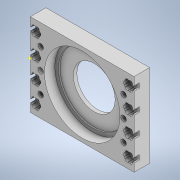
# Autodesk Inventor part: BearingBlock
Saved by Autodesk Inventor 2020 (Build 240168000, 168)
## iProperties
Created: 2020-01-26
Part Number: BearingBlock
Material: Generic
Document SubType Name: Modeling
Designer: srini
Density: 1 g/cm^3
Appearance: Default
Author: srini
Autodesk Inventor part; units mm, degrees
ref_plane "YZ Plane" through (0, 0, 0) normal (1, 0, 0) x (0, 1, 0)
ref_plane "XZ Plane" through (0, 0, 0) normal (0, 1, 0) x (-1, 0, 0)
ref_plane "XY Plane" through (0, 0, 0) normal (0, 0, 1) x (1, 0, 0)
sketch "Sketch1" plane through (0, 0, 0) normal (1, 0, 0) x (0, 1, 0)
  line L0 (43.9796, 9.0546) -> (-57.6204, 9.0546)
  line L1 (-57.6204, 9.0546) -> (-57.6204, -9.9954)
  line L2 (-57.6204, -9.9954) -> (43.9796, -9.9954)
  line L3 (43.9796, -9.9954) -> (43.9796, 9.0546)
  point P0 (0, 0)
  dimension "d0" = 19.05
  dimension "d1" = 101.6
  constraints: 8 end point, 2 parallel, 1 horizontal, 1 perpendicular
  measures "d0" distance of L2.end L0.start
  measures "d1" distance of L0.start L0.end
extrude "Extrusion1" add sketch "Sketch1" along normal blind 127
sketch "Sketch2" plane through (0, -57.6204, 9.0546) normal (0, 0, 1) x (1, 0, 0)
  circle A0 centre (63.5, 50.8) radius 25.6
  line L0 (0, 101.6) -> (0, 0) projected
  line L1 (0, 0) -> (127, 0) projected
  point P0 (0, 57.6204)
  dimension "d4" = 63.5
  dimension "d5" = 50.8
  dimension "d6" = 51.2
  constraints: 1 centre point
  measures "d4" distance from line of A0.centre L0
  measures "d5" distance from line of A0.centre L1
  measures "d6" diameter of A0
extrude "Extrusion2" cut sketch "Sketch2" against normal through all
sketch "Sketch3" plane through (0, -57.6204, 9.0546) normal (0, 0, 1) x (1, 0, 0)
  circle A0 centre (63.5, 50.8) radius 25.6 projected
  circle A1 centre (63.5, 50.8) radius 41.91
  point P0 (0, 57.6204)
  dimension "d9" = 83.82
  constraints: 1 centre point, 1 coincident
  measures "d9" diameter of A1
extrude "Extrusion3" cut sketch "Sketch3" against normal blind 14.7 contours A0 | A1
sketch "Sketch5" plane through (0, -57.6204, 9.0546) normal (0, 0, 1) x (1, 0, 0)
  circle A0 centre (63.5, 50.8) radius 25.6 projected
  circle A1 centre (63.5, 50.8) radius 46.2375
  point P0 (0, 57.6204)
  dimension "d13" = 92.475
  constraints: 1 centre point, 1 coincident
  measures "d13" diameter of A1
extrude "Extrusion4" cut sketch "Sketch5" against normal blind 12.7 contours A0 | A1
sketch "Sketch6" plane through (0, -57.6204, 9.0546) normal (0, 0, 1) x (1, 0, 0)
  circle A0 centre (6.35, 88.9) radius 3.3734
  line L0 (0, 101.6) -> (127, 101.6) projected
  line L1 (0, 101.6) -> (0, 0) projected
  circle A1 centre (120.65, 88.9) radius 3.3734
  circle A2 centre (6.35, 63.5) radius 3.3734
  circle A3 centre (120.65, 63.5) radius 3.3734
  circle A4 centre (6.35, 38.1) radius 3.3734
  circle A5 centre (120.65, 38.1) radius 3.3734
  circle A6 centre (6.35, 12.7) radius 3.3734
  circle A7 centre (120.65, 12.7) radius 3.3734
  dimension "d18" = 114.3
  dimension "d21" = 25.4
  dimension "d24" = 6.7469
  dimension "d25" = 12.7
  dimension "d26" = 6.35
  constraints: 8 centre point, 1 horizontal, 1 vertical, 14 other
  measures "d18" distance of A0.centre A1.centre
  measures "d21" distance of A0.centre A2.centre
  measures "d24" diameter of A0
  measures "d25" distance from line of A0.centre L0
  measures "d26" distance from line of A0.centre L1
extrude "Extrusion5" cut sketch "Sketch6" against normal through all
sketch "Sketch7" plane through (0, -57.6204, 9.0546) normal (0, 0, 1) x (1, 0, 0)
  circle A0 centre (6.35, 88.9) radius 3.3734 projected
  line L0 (3.0266, 94.6562) -> (9.6734, 94.6562)
  line L1 (9.6734, 94.6562) -> (12.9967, 88.9)
  line L2 (12.9967, 88.9) -> (9.6734, 83.1437)
  line L3 (9.6734, 83.1437) -> (3.0266, 83.1437)
  line L4 (3.0266, 83.1437) -> (-0.2967, 88.9)
  line L5 (-0.2967, 88.9) -> (3.0266, 94.6562)
  point P0 (0, 57.6204)
  dimension "d29" = 11.5125
  constraints: 12 end point, 1 coincident, 1 horizontal, 13 other
  measures "d29" distance between parallel lines of L3 L0
extrude "Extrusion6" cut sketch "Sketch7" against normal blind 6.35 contours A0 | L0 L1 L2 L3 L4 L5
sketch "Sketch8" plane through (0, -57.6204, 9.0546) normal (0, 0, 1) x (1, 0, 0)
  circle A0 centre (6.35, 88.9) radius 3.3734 projected
  line L0 (4.1379, 92.7315) -> (8.5621, 92.7315)
  line L1 (8.5621, 92.7315) -> (10.7742, 88.9)
  line L2 (10.7742, 88.9) -> (8.5621, 85.0685)
  line L3 (8.5621, 85.0685) -> (4.1379, 85.0685)
  line L4 (4.1379, 85.0685) -> (1.9258, 88.9)
  line L5 (1.9258, 88.9) -> (4.1379, 92.7315)
  circle A1 centre (4.1379, 92.7315) radius 2.2225
  circle A2 centre (8.5621, 92.7315) radius 2.2225
  circle A3 centre (10.7742, 88.9) radius 2.2225
  circle A4 centre (8.5621, 85.0685) radius 2.2225
  circle A5 centre (4.1379, 85.0685) radius 2.2225
  circle A6 centre (1.9258, 88.9) radius 2.2225
  point P0 (0, 57.6204)
  point P1 (3.0266, 94.6562)
  point P2 (6.35, 92.946)
  point P3 (2.846, 90.923)
  point P4 (2.846, 86.877)
  point P5 (6.35, 84.854)
  point P6 (9.854, 86.877)
  point P7 (9.854, 90.923)
  dimension "d33" = 4.445
  constraints: 12 end point, 7 coincident, 5 centre point, 3 equal radius, 1 horizontal, 18 other
extrude "Extrusion7" cut sketch "Sketch8" against normal blind 6.35
fillet "Fillet1" radius 1.5875 12 edges at (5.2491, 37.0359, 5.8796) (7.4509, 37.0359, 5.8796) (10.7846, 35.1111, 5.8796) (11.8855, 33.2044, 5.8796) (11.8855, 29.3549, 5.8796) (10.7846, 27.4481, 5.8796) (7.4509, 25.5234, 5.8796) (5.2491, 25.5234, 5.8796) (1.9154, 27.4481, 5.8796) (0.8145, 29.3549, 5.8796) (0.8145, 33.2044, 5.8796) (1.9154, 35.1111, 5.8796)
pattern_linear "Rectangular Pattern1" count 4 spacing 25.4 along (0, -1, 0) count 2 spacing 114.3 along (1, 0, 0) of "Extrusion7", "Extrusion6", "Fillet1"
sketch "Sketch9" plane through (0, 43.9796, 9.0546) normal (0, 0, 1) x (1, 0, 0)
  point P0 (0, -43.9796)
sketch "Sketch10" plane through (0, 43.9796, 9.0546) normal (0, 0, 1) x (1, 0, 0)
  circle A0 centre (12.7, -25.4) radius 3.3734
  circle A1 centre (63.5, -50.8) radius 25.6 projected
  line L0 (0, 0) -> (127, 0) projected
  circle A2 centre (6.35, -12.7) radius 3.3734 projected
  line L1 (0, 0) -> (0, -11.5905) projected
  circle A3 centre (12.7, -50.8) radius 3.3734
  circle A4 centre (12.7, -76.2) radius 3.3734
  circle A5 centre (114.3, -25.4) radius 3.3734
  circle A6 centre (114.3, -50.8) radius 3.3734
  circle A7 centre (114.3, -76.2) radius 3.3734
  point P0 (0, -43.9796)
  dimension "d43" = 50.8
  dimension "d44" = 25.4
  dimension "d47" = 25.4
  dimension "d50" = 101.6
  constraints: 6 centre point, 1 equal radius, 1 horizontal, 1 vertical, 10 other
  measures "d43" horizontal distance of A1.centre A0.centre
  measures "d44" distance from line of A0.centre L0
  measures "d47" distance of A0.centre A3.centre
  measures "d50" distance of A0.centre A5.centre
extrude "Extrusion8" cut sketch "Sketch10" against normal through all contours A0 | A2 | A3 | A4 | A5 | A6 | A7
fillet "Fillet2" radius 1.5875 16 edges at (0, 32.3891, 5.8796) (0, 30.1701, 5.8796) (0, 6.9891, 5.8796) (0, 4.7701, 5.8796) (0, -18.4109, 5.8796) (0, -20.6299, 5.8796) (0, -43.8109, 5.8796) (0, -46.0299, 5.8796) (127, -46.0299, 5.8796) (127, -43.8109, 5.8796) (127, -20.6299, 5.8796) (127, -18.4109, 5.8796) (127, 4.7701, 5.8796) (127, 6.9891, 5.8796) (127, 30.1701, 5.8796) (127, 32.3891, 5.8796)
equation "\"d4\" = 0.5 * d2"
equation "\"d42\" = d18"
equation "\"d2\" = 127"
body "Solid1"
